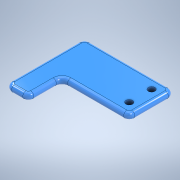
# Autodesk Inventor part: CableHook
Saved by Autodesk Inventor 2022 (Build 260153000, 153)
## iProperties
Created: 2022-02-22
Part Number: CableHook
Material: Generic
Document SubType Name: Modeling
Designer: Jorian Brusind
Density: 1 g/cm^3
Appearance: Cyan
Author: Jorian Brusind
Autodesk Inventor part; units mm, degrees
ref_plane "YZ Plane" through (0, 0, 0) normal (1, 0, 0) x (0, 1, 0)
ref_plane "XZ Plane" through (0, 0, 0) normal (0, 1, 0) x (-1, 0, 0)
ref_plane "XY Plane" through (0, 0, 0) normal (0, 0, 1) x (1, 0, 0)
sketch "Sketch1" plane through (0, 0, 0) normal (0, 1, 0) x (-1, 0, 0)
  line L0 (0, 0) -> (80, 0)
  line L1 (80, 0) -> (80, -40)
  line L2 (80, -40) -> (0, -40)
  line L3 (0, -40) -> (0, 0)
  line L4 (0, 0) -> (10, 0)
  line L5 (10, 0) -> (10, -10)
  line L6 (10, -10) -> (10, -30)
  circle A0 centre (10, -10) radius 3
  circle A1 centre (10, -30) radius 3
  line L7 (80, 0) -> (60, 0)
  line L8 (60, 0) -> (60, 30)
  line L9 (60, 30) -> (80, 30)
  line L10 (80, 30) -> (80, 0)
  dimension "d0" = 80
  dimension "d1" = 40
  dimension "d2" = 10
  dimension "d3" = 10
  dimension "d4" = 20
  dimension "d5" = 6
  dimension "d6" = 6
  dimension "d28" = 20
  dimension "d29" = 30
  constraints: 22 end point, 4 parallel, 3 perpendicular, 2 centre point, 2 coincident, 2 horizontal, 1 point on line, 1 vertical
  measures "d0" distance of L1.end L2.end
  measures "d1" distance of L0.end L1.end
  measures "d2" distance of L0.start L4.end
  measures "d3" distance of L4.end L5.end
  measures "d4" distance of L5.end L6.end
  measures "d5" diameter of A0
  measures "d6" diameter of A1
  measures "d28" distance of L8.end L9.end
  measures "d29" distance of L7.end L8.end
extrude "Extrusion1" add sketch "Sketch1" along normal blind 6
fillet "Fillet5" radius 5 6 edges at (-60, 3, 0) (-60, 3, 30) (-80, 3, 30) (0, 3, 0) (0, 3, -40) (-80, 3, -40)
fillet "Fillet6" radius 3 24 edges at (-1.4645, 6, -1.4645) (0, 6, -20) (-1.4645, 6, -38.5355) (-40, 6, -40) (-78.5355, 6, -38.5355) (-80, 6, -5) (-78.5355, 6, 28.5355) (-70, 6, 30) (-61.4645, 6, 28.5355) (-60, 6, 15) (-58.5355, 6, 1.4645) (-30, 6, 0) (-1.4645, 0, -1.4645) (0, 0, -20) (-1.4645, 0, -38.5355) (-40, 0, -40) (-78.5355, 0, -38.5355) (-80, 0, -5) (-78.5355, 0, 28.5355) (-70, 0, 30) (-61.4645, 0, 28.5355) (-60, 0, 15) (-58.5355, 0, 1.4645) (-30, 0, 0)
body "Solid1"
